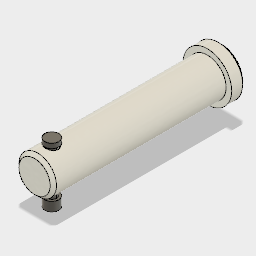
F3Z - Bras de rappel (Autodesk Fusion 360 archive; units mm, degrees)
design "0.175.4147 - Axe d'articulation avec tête 12-55 type B"
Autodesk Fusion 360 part; units mm, degrees
sketch "Sketch1" plane through (0, 0, 0) normal (0, 0, 1) x (1, 0, 0)
  circle A0 centre (0, 0) radius 6
  dimension "d1" = 12
  measures "d1" diameter of A0
extrude "Extrude1" add sketch "Sketch1" along normal blind 55 makes body 1
chamfer "Chamfer1" distance 1 angle 45 1 edges at (-5.594, -2.1697, 55) on bodies 1
sketch "Sketch2" plane through (0, 0, 0) normal (0, 0, -1) x (-1, 0, 0)
  circle A0 centre (0, 0) radius 6
  circle A1 centre (0, 0) radius 7.75
  dimension "d5" = 15.5
  measures "d5" diameter of A1
extrude "Extrude2" add sketch "Sketch2" along normal blind 4.5 contours A0 | A1 bodies 1
chamfer "Chamfer2" distance 1 angle 45 1 edges at (7.2255, -2.8025, -4.5) on bodies 1
sketch "Sketch3" plane through (0, 0, 0) normal (0, 1, 0) x (1, 0, 0)
  line L0 (-6, -54) -> (6, -54) construction
  line L1 (-6, -49.5) -> (6, -49.5) construction
  line L2 (0, -54) -> (0, -49.5) construction
  circle A0 centre (0, -49.5) radius 2
  dimension "d9" = 4.5
  dimension "d10" = 4
  measures "d10" diameter of A0
extrude "Extrude3" cut sketch "Sketch3" along normal through all and the other way through all bodies 1
sketch "Sketch4" plane through (0, 0, 0) normal (0, 1, 0) x (1, 0, 0)
  spline S0 degree 3 poles (1.5, -49.5) (1.5, -49.3138) (1.4604, -49.1052) (1.385, -48.924) (1.3095, -48.7425) (1.1904, -48.5691) (1.0607, -48.4393) (0.931, -48.3096) (0.7575, -48.1905) (0.576, -48.115) (0.3947, -48.0396) (0.186, -48) (0, -48) (-0.186, -48) (-0.3947, -48.0396) (-0.576, -48.115) (-0.7575, -48.1905) (-0.931, -48.3096) (-1.0607, -48.4393) (-1.1904, -48.5691) (-1.3095, -48.7425) (-1.385, -48.924) (-1.4604, -49.1052) (-1.5, -49.3138) (-1.5, -49.5) (-1.5, -49.6862) (-1.4604, -49.8948) (-1.385, -50.076) (-1.3095, -50.2575) (-1.1904, -50.4309) (-1.0607, -50.5607) (-0.931, -50.6904) (-0.7575, -50.8095) (-0.576, -50.885) (-0.3947, -50.9604) (-0.186, -51) (0, -51) (0.186, -51) (0.3947, -50.9604) (0.576, -50.885) (0.7575, -50.8095) (0.931, -50.6904) (1.0607, -50.5607) (1.1904, -50.4309) (1.3095, -50.2575) (1.385, -50.076) (1.4604, -49.8948) (1.5, -49.6862) (1.5, -49.5) knots 0.60776 0.60776 0.60776 0.60776 0.683748 0.683748 0.683748 0.759735 0.759735 0.759735 0.835688 0.835688 0.835688 0.91164 0.91164 0.91164 0.987593 0.987593 0.987593 1.063545 1.063545 1.063545 1.139533 1.139533 1.139533 1.21552 1.21552 1.21552 1.291508 1.291508 1.291508 1.367496 1.367496 1.367496 1.443448 1.443448 1.443448 1.5194 1.5194 1.5194 1.595353 1.595353 1.595353 1.671305 1.671305 1.671305 1.747293 1.747293 1.747293 1.82328 1.82328 1.82328 1.82328
  line L0 (0, -68) -> (8.4815, -68)
  spline S1 degree 3 poles (2, -49.5) (2, -49.2467) (1.949, -48.978) (1.7443, -48.4859) (1.5907, -48.2623) (1.2378, -47.9093) (1.0142, -47.7557) (0.5219, -47.551) (0.2532, -47.5) (-0.2532, -47.5) (-0.5219, -47.551) (-1.0142, -47.7557) (-1.2378, -47.9093) (-1.5907, -48.2623) (-1.7443, -48.4859) (-1.949, -48.978) (-2, -49.2467) (-2, -49.5) (-2, -49.7533) (-1.949, -50.022) (-1.7443, -50.5141) (-1.5907, -50.7377) (-1.2378, -51.0907) (-1.0142, -51.2443) (-0.5219, -51.449) (-0.2532, -51.5) (0.2532, -51.5) (0.5219, -51.449) (1.0142, -51.2443) (1.2378, -51.0907) (1.5907, -50.7377) (1.7443, -50.5141) (1.949, -50.022) (2, -49.7533) (2, -49.5) knots 0.60776 0.60776 0.60776 0.60776 0.683748 0.683748 0.759735 0.759735 0.835688 0.835688 0.91164 0.91164 0.987593 0.987593 1.063545 1.063545 1.139533 1.139533 1.21552 1.21552 1.21552 1.291508 1.291508 1.367496 1.367496 1.443448 1.443448 1.5194 1.5194 1.595353 1.595353 1.671305 1.671305 1.747293 1.747293 1.82328 1.82328 1.82328 1.82328
  spline S2 degree 3 poles (-2, -49.5) (-2, -49.2467) (-1.949, -48.978) (-1.7443, -48.4859) (-1.5907, -48.2623) (-1.2378, -47.9093) (-1.0142, -47.7557) (-0.5219, -47.551) (-0.2532, -47.5) (0.2532, -47.5) (0.5219, -47.551) (1.0142, -47.7557) (1.2378, -47.9093) (1.5907, -48.2623) (1.7443, -48.4859) (1.949, -48.978) (2, -49.2467) (2, -49.7533) (1.949, -50.022) (1.7443, -50.5141) (1.5907, -50.7377) (1.2378, -51.0907) (1.0142, -51.2443) (0.5219, -51.449) (0.2532, -51.5) (-0.2532, -51.5) (-0.5219, -51.449) (-1.0142, -51.2443) (-1.2378, -51.0907) (-1.5907, -50.7377) (-1.7443, -50.5141) (-1.949, -50.022) (-2, -49.7533) (-2, -49.5) knots 0 0 0 0 0.075988 0.075988 0.151975 0.151975 0.227928 0.227928 0.30388 0.30388 0.379832 0.379832 0.455785 0.455785 0.531772 0.531772 0.60776 0.60776 0.683748 0.683748 0.759735 0.759735 0.835688 0.835688 0.91164 0.91164 0.987593 0.987593 1.063545 1.063545 1.139533 1.139533 1.21552 1.21552 1.21552 1.21552
extrude "Extrude4" add sketch "Sketch4" along normal blind 8 and the other way blind 11 separate body contours S0 makes body 2
sketch "Sketch5" plane through (0, 8, 0) normal (0, 1, 0) x (-1, 0, 0)
  spline S0 degree 3 poles (1.5, -49.5) (1.5, -49.3138) (1.4604, -49.1052) (1.385, -48.924) (1.3095, -48.7425) (1.1904, -48.5691) (1.0607, -48.4393) (0.931, -48.3096) (0.7575, -48.1905) (0.576, -48.115) (0.3947, -48.0396) (0.186, -48) (0, -48) (-0.186, -48) (-0.3947, -48.0396) (-0.576, -48.115) (-0.7575, -48.1905) (-0.931, -48.3096) (-1.0607, -48.4393) (-1.1904, -48.5691) (-1.3095, -48.7425) (-1.385, -48.924) (-1.4604, -49.1052) (-1.5, -49.3138) (-1.5, -49.5) (-1.5, -49.6862) (-1.4604, -49.8948) (-1.385, -50.076) (-1.3095, -50.2575) (-1.1904, -50.4309) (-1.0607, -50.5607) (-0.931, -50.6904) (-0.7575, -50.8095) (-0.576, -50.885) (-0.3947, -50.9604) (-0.186, -51) (0, -51) (0.186, -51) (0.3947, -50.9604) (0.576, -50.885) (0.7575, -50.8095) (0.931, -50.6904) (1.0607, -50.5607) (1.1904, -50.4309) (1.3095, -50.2575) (1.385, -50.076) (1.4604, -49.8948) (1.5, -49.6862) (1.5, -49.5) knots 0.60776 0.60776 0.60776 0.60776 0.683748 0.683748 0.683748 0.759735 0.759735 0.759735 0.835688 0.835688 0.835688 0.91164 0.91164 0.91164 0.987593 0.987593 0.987593 1.063545 1.063545 1.063545 1.139533 1.139533 1.139533 1.21552 1.21552 1.21552 1.291508 1.291508 1.291508 1.367496 1.367496 1.367496 1.443448 1.443448 1.443448 1.5194 1.5194 1.5194 1.595353 1.595353 1.595353 1.671305 1.671305 1.671305 1.747293 1.747293 1.747293 1.82328 1.82328 1.82328 1.82328
  spline S1 degree 3 poles (-1.5, 49.5) (-1.5, 49.3138) (-1.4604, 49.1052) (-1.385, 48.924) (-1.3095, 48.7425) (-1.1904, 48.5691) (-1.0607, 48.4393) (-0.931, 48.3096) (-0.7575, 48.1905) (-0.576, 48.115) (-0.3947, 48.0396) (-0.186, 48) (0, 48) (0.186, 48) (0.3947, 48.0396) (0.576, 48.115) (0.7575, 48.1905) (0.931, 48.3096) (1.0607, 48.4393) (1.1904, 48.5691) (1.3095, 48.7425) (1.385, 48.924) (1.4604, 49.1052) (1.5, 49.3138) (1.5, 49.5) (1.5, 49.6862) (1.4604, 49.8948) (1.385, 50.076) (1.3095, 50.2575) (1.1904, 50.4309) (1.0607, 50.5607) (0.931, 50.6904) (0.7575, 50.8095) (0.576, 50.885) (0.3947, 50.9604) (0.186, 51) (0, 51) (-0.186, 51) (-0.3947, 50.9604) (-0.576, 50.885) (-0.7575, 50.8095) (-0.931, 50.6904) (-1.0607, 50.5607) (-1.1904, 50.4309) (-1.3095, 50.2575) (-1.385, 50.076) (-1.4604, 49.8948) (-1.5, 49.6862) (-1.5, 49.5) knots 0.60776 0.60776 0.60776 0.60776 0.683748 0.683748 0.683748 0.759735 0.759735 0.759735 0.835688 0.835688 0.835688 0.91164 0.91164 0.91164 0.987593 0.987593 0.987593 1.063545 1.063545 1.063545 1.139533 1.139533 1.139533 1.21552 1.21552 1.21552 1.291508 1.291508 1.291508 1.367496 1.367496 1.367496 1.443448 1.443448 1.443448 1.5194 1.5194 1.5194 1.595353 1.595353 1.595353 1.671305 1.671305 1.671305 1.747293 1.747293 1.747293 1.82328 1.82328 1.82328 1.82328 construction
  spline S2 degree 3 poles (-1.5, 49.5) (-1.5, 49.6862) (-1.4604, 49.8948) (-1.385, 50.076) (-1.3095, 50.2575) (-1.1904, 50.4309) (-1.0607, 50.5607) (-0.931, 50.6904) (-0.7575, 50.8095) (-0.576, 50.885) (-0.3947, 50.9604) (-0.186, 51) (0, 51) (0.186, 51) (0.3947, 50.9604) (0.576, 50.885) (0.7575, 50.8095) (0.931, 50.6904) (1.0607, 50.5607) (1.1904, 50.4309) (1.3095, 50.2575) (1.385, 50.076) (1.4604, 49.8948) (1.5, 49.6862) (1.5, 49.5) (1.5, 49.3138) (1.4604, 49.1052) (1.385, 48.924) (1.3095, 48.7425) (1.1904, 48.5691) (1.0607, 48.4393) (0.931, 48.3096) (0.7575, 48.1905) (0.576, 48.115) (0.3947, 48.0396) (0.186, 48) (0, 48) (-0.186, 48) (-0.3947, 48.0396) (-0.576, 48.115) (-0.7575, 48.1905) (-0.931, 48.3096) (-1.0607, 48.4393) (-1.1904, 48.5691) (-1.3095, 48.7425) (-1.385, 48.924) (-1.4604, 49.1052) (-1.5, 49.3138) (-1.5, 49.5) knots -1.82328 -1.82328 -1.82328 -1.82328 -1.747293 -1.747293 -1.747293 -1.671305 -1.671305 -1.671305 -1.595353 -1.595353 -1.595353 -1.5194 -1.5194 -1.5194 -1.443448 -1.443448 -1.443448 -1.367496 -1.367496 -1.367496 -1.291508 -1.291508 -1.291508 -1.21552 -1.21552 -1.21552 -1.139533 -1.139533 -1.139533 -1.063545 -1.063545 -1.063545 -0.987593 -0.987593 -0.987593 -0.91164 -0.91164 -0.91164 -0.835688 -0.835688 -0.835688 -0.759735 -0.759735 -0.759735 -0.683748 -0.683748 -0.683748 -0.60776 -0.60776 -0.60776 -0.60776 construction
  circle A0 centre (0, 49.5) radius 2.25
  spline S3 degree 3 poles (2, -49.5) (2, -49.2467) (1.949, -48.978) (1.7443, -48.4859) (1.5907, -48.2623) (1.2378, -47.9093) (1.0142, -47.7557) (0.5219, -47.551) (0.2532, -47.5) (-0.2532, -47.5) (-0.5219, -47.551) (-1.0142, -47.7557) (-1.2378, -47.9093) (-1.5907, -48.2623) (-1.7443, -48.4859) (-1.949, -48.978) (-2, -49.2467) (-2, -49.5) (-2, -49.7533) (-1.949, -50.022) (-1.7443, -50.5141) (-1.5907, -50.7377) (-1.2378, -51.0907) (-1.0142, -51.2443) (-0.5219, -51.449) (-0.2532, -51.5) (0.2532, -51.5) (0.5219, -51.449) (1.0142, -51.2443) (1.2378, -51.0907) (1.5907, -50.7377) (1.7443, -50.5141) (1.949, -50.022) (2, -49.7533) (2, -49.5) knots 0.60776 0.60776 0.60776 0.60776 0.683748 0.683748 0.759735 0.759735 0.835688 0.835688 0.91164 0.91164 0.987593 0.987593 1.063545 1.063545 1.139533 1.139533 1.21552 1.21552 1.21552 1.291508 1.291508 1.367496 1.367496 1.443448 1.443448 1.5194 1.5194 1.595353 1.595353 1.671305 1.671305 1.747293 1.747293 1.82328 1.82328 1.82328 1.82328
  spline S4 degree 3 poles (-2, -49.5) (-2, -49.2467) (-1.949, -48.978) (-1.7443, -48.4859) (-1.5907, -48.2623) (-1.2378, -47.9093) (-1.0142, -47.7557) (-0.5219, -47.551) (-0.2532, -47.5) (0.2532, -47.5) (0.5219, -47.551) (1.0142, -47.7557) (1.2378, -47.9093) (1.5907, -48.2623) (1.7443, -48.4859) (1.949, -48.978) (2, -49.2467) (2, -49.7533) (1.949, -50.022) (1.7443, -50.5141) (1.5907, -50.7377) (1.2378, -51.0907) (1.0142, -51.2443) (0.5219, -51.449) (0.2532, -51.5) (-0.2532, -51.5) (-0.5219, -51.449) (-1.0142, -51.2443) (-1.2378, -51.0907) (-1.5907, -50.7377) (-1.7443, -50.5141) (-1.949, -50.022) (-2, -49.7533) (-2, -49.5) knots 0 0 0 0 0.075988 0.075988 0.151975 0.151975 0.227928 0.227928 0.30388 0.30388 0.379832 0.379832 0.455785 0.455785 0.531772 0.531772 0.60776 0.60776 0.683748 0.683748 0.759735 0.759735 0.835688 0.835688 0.91164 0.91164 0.987593 0.987593 1.063545 1.063545 1.139533 1.139533 1.21552 1.21552 1.21552 1.21552
  spline S5 degree 3 poles (1.5, 49.5) (1.4997, 49.5291) (1.499, 49.5582) (1.4876, 49.7407) (1.4443, 49.9464) (1.2744, 50.3221) (1.1579, 50.4635) (1.0607, 50.5607) (0.9778, 50.6435) (0.881, 50.7184) (0.6163, 50.8807) (0.5167, 50.9099) (0.2655, 50.9873) (0.0596, 51.0123) (-0.2987, 50.9775) (-0.5139, 50.9246) (-0.8641, 50.7393) (-1.0281, 50.6108) (-1.2584, 50.3304) (-1.3708, 50.1429) (-1.4869, 49.7672) (-1.5123, 49.5612) (-1.478, 49.2046) (-1.4256, 48.9888) (-1.2414, 48.6391) (-1.1133, 48.4745) (-0.8077, 48.2224) (-0.6295, 48.1258) (-0.2761, 48.0151) (-0.0693, 47.988) (0.2839, 48.0201) (0.5004, 48.0708) (0.8431, 48.2475) (1.0118, 48.3739) (1.2827, 48.6947) (1.368, 48.8621) (1.4579, 49.1311) (1.4977, 49.3165) (1.5, 49.5) knots -0.080744 -0.080744 -0.080744 -0.080744 -0.074519 -0.074519 -0.041241 -0.041241 0 0 0 0.035143 0.035143 0.092639 0.092639 0.246463 0.246463 0.37223 0.37223 0.489793 0.489793 0.586811 0.586811 0.67816 0.67816 0.752062 0.752062 0.820566 0.820566 0.888592 0.888592 0.958337 0.958337 1.013363 1.013363 1.062684 1.062684 1.116599 1.116599 1.155794 1.155794 1.155794 1.155794
  spline S6 degree 3 poles (2, 49.5) (2, 49.2467) (1.949, 48.978) (1.7443, 48.4859) (1.5907, 48.2623) (1.2378, 47.9093) (1.0142, 47.7557) (0.5219, 47.551) (0.2532, 47.5) (-0.2532, 47.5) (-0.5219, 47.551) (-1.0142, 47.7557) (-1.2378, 47.9093) (-1.5907, 48.2623) (-1.7443, 48.4859) (-1.949, 48.978) (-2, 49.2467) (-2, 49.5) (-2, 49.7533) (-1.949, 50.022) (-1.7443, 50.5141) (-1.5907, 50.7377) (-1.2378, 51.0907) (-1.0142, 51.2443) (-0.5219, 51.449) (-0.2532, 51.5) (0.2532, 51.5) (0.5219, 51.449) (1.0142, 51.2443) (1.2378, 51.0907) (1.5907, 50.7377) (1.7443, 50.5141) (1.949, 50.022) (2, 49.7533) (2, 49.5) knots 0.60776 0.60776 0.60776 0.60776 0.683748 0.683748 0.759735 0.759735 0.835688 0.835688 0.91164 0.91164 0.987593 0.987593 1.063545 1.063545 1.139533 1.139533 1.21552 1.21552 1.21552 1.291508 1.291508 1.367496 1.367496 1.443448 1.443448 1.5194 1.5194 1.595353 1.595353 1.671305 1.671305 1.747293 1.747293 1.82328 1.82328 1.82328 1.82328
  spline S7 degree 3 poles (-2, 49.5) (-2, 49.2467) (-1.949, 48.978) (-1.7443, 48.4859) (-1.5907, 48.2623) (-1.2378, 47.9093) (-1.0142, 47.7557) (-0.5219, 47.551) (-0.2532, 47.5) (0.2532, 47.5) (0.5219, 47.551) (1.0142, 47.7557) (1.2378, 47.9093) (1.5907, 48.2623) (1.7443, 48.4859) (1.949, 48.978) (2, 49.2467) (2, 49.7533) (1.949, 50.022) (1.7443, 50.5141) (1.5907, 50.7377) (1.2378, 51.0907) (1.0142, 51.2443) (0.5219, 51.449) (0.2532, 51.5) (-0.2532, 51.5) (-0.5219, 51.449) (-1.0142, 51.2443) (-1.2378, 51.0907) (-1.5907, 50.7377) (-1.7443, 50.5141) (-1.949, 50.022) (-2, 49.7533) (-2, 49.5) knots 0 0 0 0 0.075988 0.075988 0.151975 0.151975 0.227928 0.227928 0.30388 0.30388 0.379832 0.379832 0.455785 0.455785 0.531772 0.531772 0.60776 0.60776 0.683748 0.683748 0.759735 0.759735 0.835688 0.835688 0.91164 0.91164 0.987593 0.987593 1.063545 1.063545 1.139533 1.139533 1.21552 1.21552 1.21552 1.21552
  dimension "d18" = 4.5
  measures "d18" diameter of A0
extrude "Extrude5" add sketch "Sketch5" against normal blind 1.5 contours A0 | S5 | S6 S7 bodies 2
sketch "Sketch6" plane through (0, -11, 0) normal (0, -1, 0) x (1, 0, 0)
  spline S0 degree 3 poles (1.5, 49.5) (1.5, 49.6862) (1.4604, 49.8948) (1.385, 50.076) (1.3095, 50.2575) (1.1904, 50.4309) (1.0607, 50.5607) (0.931, 50.6904) (0.7575, 50.8095) (0.576, 50.885) (0.3947, 50.9604) (0.186, 51) (0, 51) (-0.186, 51) (-0.3947, 50.9604) (-0.576, 50.885) (-0.7575, 50.8095) (-0.931, 50.6904) (-1.0607, 50.5607) (-1.1904, 50.4309) (-1.3095, 50.2575) (-1.385, 50.076) (-1.4604, 49.8948) (-1.5, 49.6862) (-1.5, 49.5) (-1.5, 49.3138) (-1.4604, 49.1052) (-1.385, 48.924) (-1.3095, 48.7425) (-1.1904, 48.5691) (-1.0607, 48.4393) (-0.931, 48.3096) (-0.7575, 48.1905) (-0.576, 48.115) (-0.3947, 48.0396) (-0.186, 48) (0, 48) (0.186, 48) (0.3947, 48.0396) (0.576, 48.115) (0.7575, 48.1905) (0.931, 48.3096) (1.0607, 48.4393) (1.1904, 48.5691) (1.3095, 48.7425) (1.385, 48.924) (1.4604, 49.1052) (1.5, 49.3138) (1.5, 49.5) knots -1.82328 -1.82328 -1.82328 -1.82328 -1.747293 -1.747293 -1.747293 -1.671305 -1.671305 -1.671305 -1.595353 -1.595353 -1.595353 -1.5194 -1.5194 -1.5194 -1.443448 -1.443448 -1.443448 -1.367496 -1.367496 -1.367496 -1.291508 -1.291508 -1.291508 -1.21552 -1.21552 -1.21552 -1.139533 -1.139533 -1.139533 -1.063545 -1.063545 -1.063545 -0.987593 -0.987593 -0.987593 -0.91164 -0.91164 -0.91164 -0.835688 -0.835688 -0.835688 -0.759735 -0.759735 -0.759735 -0.683748 -0.683748 -0.683748 -0.60776 -0.60776 -0.60776 -0.60776 construction
  spline S1 degree 3 poles (1.5, 49.5) (1.5, 49.6862) (1.4604, 49.8948) (1.385, 50.076) (1.3095, 50.2575) (1.1904, 50.4309) (1.0607, 50.5607) (0.931, 50.6904) (0.7575, 50.8095) (0.576, 50.885) (0.3947, 50.9604) (0.186, 51) (0, 51) (-0.186, 51) (-0.3947, 50.9604) (-0.576, 50.885) (-0.7575, 50.8095) (-0.931, 50.6904) (-1.0607, 50.5607) (-1.1904, 50.4309) (-1.3095, 50.2575) (-1.385, 50.076) (-1.4604, 49.8948) (-1.5, 49.6862) (-1.5, 49.5) (-1.5, 49.3138) (-1.4604, 49.1052) (-1.385, 48.924) (-1.3095, 48.7425) (-1.1904, 48.5691) (-1.0607, 48.4393) (-0.931, 48.3096) (-0.7575, 48.1905) (-0.576, 48.115) (-0.3947, 48.0396) (-0.186, 48) (0, 48) (0.186, 48) (0.3947, 48.0396) (0.576, 48.115) (0.7575, 48.1905) (0.931, 48.3096) (1.0607, 48.4393) (1.1904, 48.5691) (1.3095, 48.7425) (1.385, 48.924) (1.4604, 49.1052) (1.5, 49.3138) (1.5, 49.5) knots -1.82328 -1.82328 -1.82328 -1.82328 -1.747293 -1.747293 -1.747293 -1.671305 -1.671305 -1.671305 -1.595353 -1.595353 -1.595353 -1.5194 -1.5194 -1.5194 -1.443448 -1.443448 -1.443448 -1.367496 -1.367496 -1.367496 -1.291508 -1.291508 -1.291508 -1.21552 -1.21552 -1.21552 -1.139533 -1.139533 -1.139533 -1.063545 -1.063545 -1.063545 -0.987593 -0.987593 -0.987593 -0.91164 -0.91164 -0.91164 -0.835688 -0.835688 -0.835688 -0.759735 -0.759735 -0.759735 -0.683748 -0.683748 -0.683748 -0.60776 -0.60776 -0.60776 -0.60776 construction
  circle A0 centre (0, 49.5) radius 2.25
  spline S2 degree 3 poles (1.5, 49.5) (1.4997, 49.5291) (1.499, 49.5582) (1.4876, 49.7407) (1.4443, 49.9464) (1.2744, 50.3221) (1.1579, 50.4635) (1.0607, 50.5607) (0.9778, 50.6435) (0.881, 50.7184) (0.6163, 50.8807) (0.5167, 50.9099) (0.2655, 50.9873) (0.0596, 51.0123) (-0.2987, 50.9775) (-0.5139, 50.9246) (-0.8641, 50.7393) (-1.0281, 50.6108) (-1.2584, 50.3304) (-1.3708, 50.1429) (-1.4869, 49.7672) (-1.5123, 49.5612) (-1.478, 49.2046) (-1.4256, 48.9888) (-1.2414, 48.6391) (-1.1133, 48.4745) (-0.8077, 48.2224) (-0.6295, 48.1258) (-0.2761, 48.0151) (-0.0693, 47.988) (0.2839, 48.0201) (0.5004, 48.0708) (0.8431, 48.2475) (1.0118, 48.3739) (1.2827, 48.6947) (1.368, 48.8621) (1.4579, 49.1311) (1.4977, 49.3165) (1.5, 49.5) knots -0.080744 -0.080744 -0.080744 -0.080744 -0.074519 -0.074519 -0.041241 -0.041241 0 0 0 0.035143 0.035143 0.092639 0.092639 0.246463 0.246463 0.37223 0.37223 0.489793 0.489793 0.586811 0.586811 0.67816 0.67816 0.752062 0.752062 0.820566 0.820566 0.888592 0.888592 0.958337 0.958337 1.013363 1.013363 1.062684 1.062684 1.116599 1.116599 1.155794 1.155794 1.155794 1.155794
  spline S3 degree 3 poles (2, 49.5) (2, 49.2467) (1.949, 48.978) (1.7443, 48.4859) (1.5907, 48.2623) (1.2378, 47.9093) (1.0142, 47.7557) (0.5219, 47.551) (0.2532, 47.5) (-0.2532, 47.5) (-0.5219, 47.551) (-1.0142, 47.7557) (-1.2378, 47.9093) (-1.5907, 48.2623) (-1.7443, 48.4859) (-1.949, 48.978) (-2, 49.2467) (-2, 49.5) (-2, 49.7533) (-1.949, 50.022) (-1.7443, 50.5141) (-1.5907, 50.7377) (-1.2378, 51.0907) (-1.0142, 51.2443) (-0.5219, 51.449) (-0.2532, 51.5) (0.2532, 51.5) (0.5219, 51.449) (1.0142, 51.2443) (1.2378, 51.0907) (1.5907, 50.7377) (1.7443, 50.5141) (1.949, 50.022) (2, 49.7533) (2, 49.5) knots 0.60776 0.60776 0.60776 0.60776 0.683748 0.683748 0.759735 0.759735 0.835688 0.835688 0.91164 0.91164 0.987593 0.987593 1.063545 1.063545 1.139533 1.139533 1.21552 1.21552 1.21552 1.291508 1.291508 1.367496 1.367496 1.443448 1.443448 1.5194 1.5194 1.595353 1.595353 1.671305 1.671305 1.747293 1.747293 1.82328 1.82328 1.82328 1.82328
  spline S4 degree 3 poles (-2, 49.5) (-2, 49.2467) (-1.949, 48.978) (-1.7443, 48.4859) (-1.5907, 48.2623) (-1.2378, 47.9093) (-1.0142, 47.7557) (-0.5219, 47.551) (-0.2532, 47.5) (0.2532, 47.5) (0.5219, 47.551) (1.0142, 47.7557) (1.2378, 47.9093) (1.5907, 48.2623) (1.7443, 48.4859) (1.949, 48.978) (2, 49.2467) (2, 49.7533) (1.949, 50.022) (1.7443, 50.5141) (1.5907, 50.7377) (1.2378, 51.0907) (1.0142, 51.2443) (0.5219, 51.449) (0.2532, 51.5) (-0.2532, 51.5) (-0.5219, 51.449) (-1.0142, 51.2443) (-1.2378, 51.0907) (-1.5907, 50.7377) (-1.7443, 50.5141) (-1.949, 50.022) (-2, 49.7533) (-2, 49.5) knots 0 0 0 0 0.075988 0.075988 0.151975 0.151975 0.227928 0.227928 0.30388 0.30388 0.379832 0.379832 0.455785 0.455785 0.531772 0.531772 0.60776 0.60776 0.683748 0.683748 0.759735 0.759735 0.835688 0.835688 0.91164 0.91164 0.987593 0.987593 1.063545 1.063545 1.139533 1.139533 1.21552 1.21552 1.21552 1.21552
  point P0 (1.5, 49.5)
  dimension "d21" = 4.5
  measures "d21" diameter of A0
extrude "Extrude6" add sketch "Sketch6" against normal blind 3 contours A0 | S2 | S3 S4 bodies 2

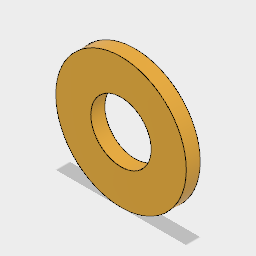
design "0.168.0152 - Rondelle M12"
Autodesk Fusion 360 part; units mm, degrees
sketch "Sketch1" plane through (0, 0, 0) normal (0, 0, 1) x (1, 0, 0)
  circle A0 centre (0, 0) radius 6
  circle A1 centre (0, 0) radius 13
  dimension "d1" = 12
  dimension "d2" = 26
  measures "d1" diameter of A0
  measures "d2" diameter of A1
extrude "Extrude1" add sketch "Sketch1" along normal blind 2.8
